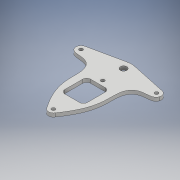
# Autodesk Inventor part: Corpo_Suporte_4_Cabos_Modelo4
Saved by Autodesk Inventor 2018 (Build 220112000, 112)
## iProperties
Created: 2021-08-09
Part Number: Corpo_Suporte_4_Cabos_Modelo4
Material: Generic
Document SubType Name: Modeling
Designer: L08619
Density: 1 g/cm^3
Appearance: Default
Author: L08619
Autodesk Inventor part; units mm, degrees
ref_plane "YZ Plane" through (0, 0, 0) normal (1, 0, 0) x (0, 1, 0)
ref_plane "XZ Plane" through (0, 0, 0) normal (0, 1, 0) x (-1, 0, 0)
ref_plane "XY Plane" through (0, 0, 0) normal (0, 0, 1) x (1, 0, 0)
sketch "Sketch2" plane through (0, 0, 0) normal (0, 0, 1) x (1, 0, 0)
  circle A0 centre (-235, 0) radius 11
  circle A1 centre (235, 0) radius 11
  circle A2 centre (0, -407.032) radius 11
  line L0 (-45, -290) -> (45, -290)
  line L1 (70, -265) -> (70, -155)
  line L2 (45, -130) -> (-45, -130)
  line L3 (-70, -155) -> (-70, -265)
  line L4 (0, -130) -> (0, -100) construction
  circle A3 centre (0, -100) radius 11
  arc A4 (-45, -130) -> (-70, -155) centre (-45, -155) ccw
  arc A5 (70, -155) -> (45, -130) centre (45, -155) ccw
  arc A6 (45, -290) -> (70, -265) centre (45, -265) ccw
  arc A7 (-70, -265) -> (-45, -290) centre (-45, -265) ccw
  line L5 (0, 0) -> (0, 30) construction
  circle A8 centre (0, 30) radius 20
  line L6 (0, 129.0435) -> (0, -459.178)
  line L7 (-241.7889, 29.2217) -> (-20, 76.6995)
  arc A9 (20, 76.6995) -> (-20, 76.6995) centre (0, -16.729) ccw
  line L8 (20, 76.6995) -> (241.7889, 29.2217)
  arc A10 (-26.5499, -421) -> (26.5499, -421) centre (0, -407.032) ccw
  arc A11 (-240.7687, 29.4401) -> (-262.9106, -11) centre (-235, 0) ccw
  arc A12 (262.9106, -11) -> (240.7687, 29.4401) centre (235, 0) ccw
  line L9 (-262.9106, -11) -> (-250, -54) construction
  line L10 (-250, -54) -> (-126, 6.6687) construction
  line L11 (-126, 6.6687) -> (-80.7749, -123) construction
  line L12 (-80.7749, -123) -> (-143, -253) construction
  line L13 (-143, -253) -> (-26.5499, -421) construction
  spline S0 degree 4 poles (-262.9106, -11) (-250, -54) (-126, 6.6687) (-80.7749, -123) (-143, -253) (-26.5499, -421) knots 1 1 1 1 1 2 3 3 3 3 3
  line L14 (262.9106, -11) -> (250, -54) construction
  line L15 (250, -54) -> (126, 6.6687) construction
  line L16 (126, 6.6687) -> (80.7749, -123) construction
  line L17 (80.7749, -123) -> (143, -253) construction
  line L18 (143, -253) -> (26.5499, -421) construction
  spline S1 degree 4 poles (262.9106, -11) (250, -54) (126, 6.6687) (80.7749, -123) (143, -253) (26.5499, -421) knots 1 1 1 1 1 2 3 3 3 3 3
  point P0 (70, -130)
  point P1 (70, -290)
  point P2 (-70, -130)
  point P3 (-17.2975, -383.8099)
  point P4 (-17.2975, -383.8099)
  dimension "d24" = 22
  dimension "d25" = 22
  dimension "d26" = 470
  dimension "d31" = 22
  dimension "d32" = 407.032
  dimension "d33" = 0
  dimension "d39" = 160
  dimension "d40" = 140
  dimension "d41" = 30
  dimension "d42" = 22
  dimension "d43" = 25
  dimension "d44" = 30
  dimension "d46" = 40
  dimension "d53" = 130
  dimension "d54" = 30
  dimension "d55" = 60
  dimension "d56" = 60
  dimension "d57" = 60
  constraints: 18 end point, 16 point on circle, 13 centre point, 10 tangent, 9 point on line, 6 coincident, 6 symmetric about line, 3 equal radius, 2 parallel, 1 horizontal, 1 horizontal alignment, 1 midpoint, 1 perpendicular, 1 vertical, 8 other
  measures "d24" diameter of A0
  measures "d25" diameter of A1
  measures "d26" distance of A0.centre A1.centre
  measures "d31" diameter of A2
  measures "d32" vertical distance of A1.centre A2.centre
  measures "d33" vertical distance of L5.start A1.centre
  measures "d39" distance of point (70, -290) point (70, -130)
  measures "d40" distance of point (70, -130) point (-70, -130)
  measures "d41" distance of L4.start L4.end
  measures "d42" diameter of A3
  measures "d43" radius of A4
  measures "d44" distance of L5.start L5.end
  measures "d46" diameter of A8
  measures "d53" distance of A3.centre A8.centre
  measures "d54" distance from line of L4.end L2
  measures "d55" diameter of A10
  measures "d56" diameter of A11
  measures "d57" diameter of A12
extrude "Extrusion1" add sketch "Sketch2" along normal mid plane 22.22 contours A2 L6 L0 A6 L1 A5 L2 A3 A8 A9 L8 A12 S1 A10 | A2 L6 A10 S0 A11 L7 A9 A8 A3 L2 A4 L3 A7 L0 | A11 L7 | L8 A12
body "Solid1"
